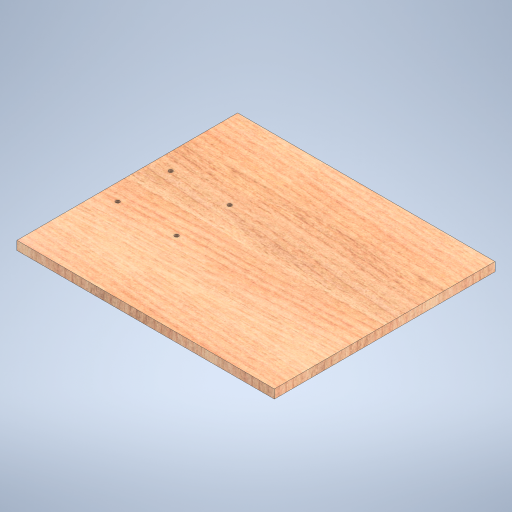
# Autodesk Inventor part: base_plates
Saved by Autodesk Inventor 2024.2 (Build 282272000, 272)
## iProperties
Created: 2022-10-18
Part Number: base_plates
Material: Wood (Birch)
Document SubType Name: Modeling
Designer: 박동준
Density: 0.55 g/cm^3
Appearance: Birch - Natural Polished
Sheet Metal Rule: Default_mm
Author: 박동준
Autodesk Inventor part; units mm, degrees
ref_plane "YZ Plane" through (0, 0, 0) normal (1, 0, 0) x (0, 1, 0)
ref_plane "XZ Plane" through (0, 0, 0) normal (0, 1, 0) x (-1, 0, 0)
ref_plane "XY Plane" through (0, 0, 0) normal (0, 0, 1) x (1, 0, 0)
sketch "Sketch7" plane through (0, 0, 0) normal (0, 1, 0) x (-1, 0, 0)
  line L0 (52.95, -150) -> (-297.05, -150)
  line L1 (-297.05, -150) -> (-297.05, 150)
  line L2 (-297.05, 150) -> (52.95, 150)
  line L3 (52.95, 150) -> (52.95, -150)
  point P0 (0, 0)
  point P1 (52.95, 0)
  dimension "d32" = 350
  dimension "d33" = 300
  dimension "d34" = 52.95
  constraints: 8 end point, 2 parallel, 1 horizontal, 1 horizontal alignment, 1 midpoint, 1 perpendicular
  measures "d32" distance of L1.end L2.end
  measures "d33" distance of L0.end L1.end
  measures "d34" distance of point (0, 0) point (52.95, 0)
extrude "Extrusion4" add sketch "Sketch7" against normal blind 12
sketch "Sketch8" plane through (0, -12, 0) normal (0, -1, 0) x (1, 0, 0)
  line L0 (54.25, -50.07) -> (54.25, 50.07) projected
  line L1 (45.95, -50.07) -> (45.95, 50.07) projected
  line L2 (-34.15, -50.07) -> (-34.15, 50.07) projected
  line L3 (-25.85, -50.07) -> (-25.85, 50.07) projected
  line L4 (-34.15, -50.07) -> (-25.85, -50.07)
  line L5 (-34.15, 50.07) -> (-25.85, 50.07)
  line L6 (45.95, 50.07) -> (54.25, 50.07)
  line L7 (45.95, -50.07) -> (54.25, -50.07)
  line L8 (-30, -50.07) -> (-30, 50.07)
  line L9 (50.1, -50.07) -> (50.1, 50.07)
  line L10 (-25.85, 0) -> (45.95, 0)
  point P0 (0, 0)
  point P1 (-30, -36.07)
  point P2 (50.1, -36.07)
  point P3 (-30, 36.07)
  point P4 (50.1, 36.07)
  dimension "d37" = 14
  constraints: 14 end point, 6 midpoint, 3 equal length, 2 point on line, 2 symmetric about line, 1 horizontal, 1 horizontal alignment
  measures "d37" distance from line of point (-30, -36.07) L4
hole "Hole3" at (-30, -12, -36.07) at (50.1, -12, -36.07) at (-30, -12, 36.07) at (50.1, -12, 36.07) direction (0, 1, 0) diameter 5.2 end through all countersink diameter 12 countersink angle 90
equation "\"TransitionRadius\" = BendRadius"
equation "\"BendRadius\" = 0.5"
body "Solid2"
